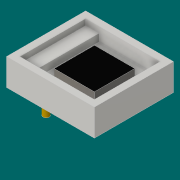
# Autodesk Inventor part: MPPC
Saved by Autodesk Inventor 2016 (Build 200138000, 138)
## iProperties
Created: 2015-08-14
Part Number: MPPC
Material: ABS Plastic
Document SubType Name: Modeling
Designer: Cosmic
Density: 1.06 g/cm^3
Appearance: Smooth - White
Author: Cosmic
Autodesk Inventor part; units mm, degrees
ref_plane "YZ Plane" through (0, 0, 0) normal (1, 0, 0) x (0, 1, 0)
ref_plane "XZ Plane" through (0, 0, 0) normal (0, 1, 0) x (-1, 0, 0)
ref_plane "XY Plane" through (0, 0, 0) normal (0, 0, 1) x (1, 0, 0)
sketch "Sketch1" plane through (0, 0, 0) normal (0, 0, 1) x (1, 0, 0)
  line L0 (-3.275, -2.95) -> (3.275, -2.95)
  line L1 (3.275, -2.95) -> (3.275, 2.95)
  line L2 (3.275, 2.95) -> (-3.275, 2.95)
  line L3 (-3.275, 2.95) -> (-3.275, -2.95)
  line L4 (-3.275, -2.95) -> (3.275, 2.95) construction
  line L5 (3.275, -2.95) -> (-3.275, 2.95) construction
  point P0 (0, 0)
  dimension "d0" = 6.55
  dimension "d1" = 5.9
  constraints: 12 end point, 2 midpoint, 2 parallel, 1 horizontal, 1 perpendicular
  measures "d0" distance of L2.end L1.end
  measures "d1" distance of L1.end L0.end
extrude "Extrusion1" add sketch "Sketch1" along normal blind 2
sketch "Sketch2" plane through (0, 0, 2) normal (0, 0, 1) x (1, 0, 0)
  line L0 (-3.275, -2.95) -> (3.275, -2.95) projected
  line L1 (3.275, -2.95) -> (3.275, 2.95) projected
  line L2 (3.275, 2.95) -> (-3.275, 2.95) projected
  line L3 (-3.275, 2.95) -> (-3.275, -2.95) projected
  line L4 (-2.775, 2.45) -> (2.775, 2.45)
  line L5 (2.775, 2.45) -> (2.775, -2.45)
  line L6 (2.775, -2.45) -> (-2.775, -2.45)
  line L7 (-2.775, -2.45) -> (-2.775, 2.45)
  point P0 (0, 0)
  dimension "d4" = 0.5
  constraints: 8 end point, 3 other
  measures "d4" distance between parallel lines of L2 L4
extrude "Extrusion2" cut sketch "Sketch2" against normal blind 1 contours L4 L5 L6 L7
sketch "Sketch3" plane through (0, 0, 1) normal (0, 0, 1) x (1, 0, 0)
  line L0 (-2.775, 2.45) -> (2.775, 2.45) projected
  line L1 (-2.775, -2.45) -> (-2.775, 2.45) projected
  line L2 (2.775, -2.45) -> (-2.775, -2.45) projected
  line L3 (2.775, 2.45) -> (2.775, -2.45) projected
  line L4 (-1.17, 1.5) -> (1.83, 1.5)
  line L5 (1.83, 1.5) -> (1.83, -1.5)
  line L6 (1.83, -1.5) -> (-1.17, -1.5)
  line L7 (-1.17, -1.5) -> (-1.17, 1.5)
  line L8 (-1.17, 1.5) -> (1.83, -1.5) construction
  line L9 (1.83, 1.5) -> (-1.17, -1.5) construction
  line L10 (-2.775, 2.45) -> (-1.775, 2.45)
  line L11 (-1.775, 2.45) -> (-1.775, -2.45)
  line L12 (-1.775, -2.45) -> (-2.775, -2.45)
  line L13 (-2.775, -2.45) -> (-2.775, 2.45)
  point P0 (0, 0)
  point P1 (0.33, 0)
  dimension "d7" = 3
  dimension "d8" = 3
  dimension "d9" = 0.33
  dimension "d10" = 0
  dimension "d11" = 1
  dimension "d13" = 0
  dimension "d14" = 0
  dimension "d15" = 0
  constraints: 20 end point, 4 parallel, 2 horizontal, 2 midpoint, 2 perpendicular
  measures "d7" distance of L5.end L6.end
  measures "d8" distance of L4.end L5.end
  measures "d9" distance of point (0, 0) point (0.33, 0)
  measures "d10" vertical distance of point (0, 0) point (0.33, 0)
  measures "d11" distance of L10.start L10.end
  measures "d13" distance between parallel lines of L0 L10
  measures "d14" distance between parallel lines of L2 L12
  measures "d15" distance between parallel lines of L1 L13
extrude "Extrusion3" add sketch "Sketch3" along normal blind 0.55 contours L0 L11 L2 L1 | L4 L5 L6 L7
sketch "Sketch4" plane through (0, 0, 0) normal (0, 0, -1) x (-1, 0, 0)
  line L0 (3.275, -2.95) -> (-3.275, -2.95) projected
  line L1 (3.275, 2.95) -> (3.275, -2.95) projected
  line L2 (-3.275, 2.95) -> (3.275, 2.95) projected
  line L3 (-3.275, -2.95) -> (-3.275, 2.95) projected
  circle A0 centre (2, 1.27) radius 0.23
  circle A1 centre (2, -1.27) radius 0.23
  line L4 (1.775, 2.45) -> (1.775, -2.45) projected
  line L5 (2, 1.27) -> (2, -1.27)
  line L6 (0, 0) -> (3.275, 0)
  point P0 (2, 0)
  dimension "d18" = 2
  dimension "d19" = 2
  dimension "d20" = 2.54
  dimension "d21" = 0.46
  dimension "d22" = 0.46
  constraints: 4 end point, 2 centre point, 2 midpoint, 1 point on line
  measures "d18" horizontal distance of L5.start L6.start
  measures "d19" horizontal distance of L6.start L5.end
  measures "d20" distance of L5.end L5.start
  measures "d21" diameter of A0
  measures "d22" diameter of A1
extrude "Extrusion4" add sketch "Sketch4" along normal blind 2 contours A0 L4 | A1 L4 | A0 L4 | L4 A1
equation "\"d0\" = MPPCHeight"
equation "\"d1\" = MPPCWidth"
equation "\"d19\" = d18"
equation "\"d22\" = d21"
equation "\"OpticalFiberDiameter\" = 1"
equation "\"OpticalFiberClearence\" = 0.15"
equation "\"SmallTrackDiameter\" = 175"
equation "\"ScintillatorEdgeClearence\" = 3"
equation "\"ScintillatorWidth\" = 145"
equation "\"ScintillatorHeight\" = 145"
equation "\"ShallowTrackDepth\" = 1.3"
equation "\"MPPCClearence\" = 0.075"
equation "\"MPPCSensorClearence\" = 1.45"
equation "\"MPPCSensorOffsett\" = 2.105"
equation "\"MPPCWidth\" = 5.9"
equation "\"MPPCHeight\" = 6.55"
equation "\"FiberEdgeOffsett\" = 5"
equation "\"MPPCDepth\" = 0"
equation "\"LongFiberAngle\" = 30deg"
equation "\"ShortFiberAngle\" = 78deg"
equation "\"LoopLargeTrackRatio\" = 1.1"
equation "\"FiberSensorClerence\" = 0.5"
equation "\"MountingScrewDepth\" = 4"
body "Solid1"
